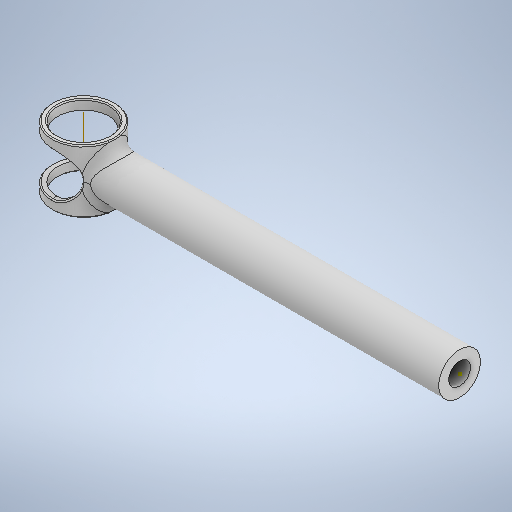
# Autodesk Inventor part: female_leg
Saved by Autodesk Inventor 2025.1 (Build 291241000, 241)
## iProperties
Created: 2024-10-31
Part Number: female_leg
Material: Generisch
Document SubType Name: Modeling
Designer: ZOMBULLI
Density: 1 g/cm^3
Appearance: Vorgabe
Author: ZOMBULLI
Autodesk Inventor part; units mm, degrees
ref_plane "YZ Plane" through (0, 0, 0) normal (1, 0, 0) x (0, 1, 0)
ref_plane "XZ Plane" through (0, 0, 0) normal (0, 1, 0) x (-1, 0, 0)
ref_plane "XY Plane" through (0, 0, 0) normal (0, 0, 1) x (1, 0, 0)
sketch "Skizze1" plane through (0, 0, 0) normal (0, 0, 1) x (1, 0, 0)
  line L0 (-34.5, 4) -> (37.5, 4)
  line L1 (37.5, 4) -> (37.5, 0)
  line L2 (37.5, 0) -> (-34.5, 0)
  line L3 (-34.5, 0) -> (-34.5, 4)
  line L4 (-48.9, 0) -> (51.9, 0) projected
  line L5 (0, 4.8) -> (0, -0.8) projected
  point P0 (0, 0)
  dimension "d0" = 72
  dimension "d1" = 4
  dimension "d2" = 0
  dimension "d3" = 37.5
  constraints: 8 end point, 2 parallel, 1 horizontal, 1 perpendicular
  measures "d0" distance of L0.start L0.end
  measures "d1" distance of L0.end L1.end
  measures "d2" distance between parallel lines of L4 L2
  measures "d3" distance between parallel lines of L1 L5
revolve "Umdrehung1" add sketch "Skizze1" angle 360 about axis through (37.5, 0, 0) along (-1, 0, 0)
sketch "Skizze2" plane through (0, 0, 0) normal (0, 0, 1) x (1, 0, 0)
  line L0 (-34.5, 4) -> (-34.5, -4) projected
  circle A0 centre (-34.5, 0) radius 6
  point P0 (0, 0)
  dimension "d5" = 12
  constraints: 1 centre point, 1 midpoint
  measures "d5" diameter of A0
extrude "Extrusion1" add sketch "Skizze2" along normal mid plane 12
fillet "Rundung1" radius 2 4 edges at (-29.3185, 3.0252, -2.6169) (-29.3186, -3.0255, -2.6166) (-29.3185, -3.0252, 2.6169) (-29.3185, 3.0252, 2.6169)
sketch "Skizze3" plane through (-34.5, 0, 6) normal (0, 0, 1) x (1, 0, 0)
  circle A0 centre (0, 0) radius 5
  point P0 (34.5, 0)
  dimension "d9" = 10
  constraints: 1 centre point
  measures "d9" diameter of A0
extrude "Extrusion2" cut sketch "Skizze3" against normal blind 15
sketch "Skizze4" plane through (0, 0, 0) normal (0, 1, 0) x (-1, 0, 0)
  line L0 (44.65, -4.15) -> (34.65, -4.15)
  line L1 (34.65, 4.15) -> (44.65, 4.15)
  line L2 (44.65, 4.15) -> (44.65, -4.15)
  arc A0 (30.5, 0) -> (34.65, -4.15) centre (34.65, 0) ccw
  arc A1 (34.65, 4.15) -> (30.5, 0) centre (34.65, 0) ccw
  line L3 (-53.715, 0) -> (59.79, 0) projected
  line L4 (30.5, 0) -> (30.5, -4.9478) construction
  line L5 (59.79, 0) -> (-53.715, 0) projected
  line L6 (29.5, 6) -> (39.5, 6) projected
  line L7 (29.5, 6) -> (29.5, -6.3947) construction
  point P0 (0, 0)
  point P1 (30.5, -2.4739)
  point P2 (30.5, 0)
  dimension "d12" = 4.15
  dimension "d13" = 8.3
  dimension "d14" = 4.15
  dimension "d15" = 1
  dimension "d16" = 10
  constraints: 10 end point, 4 point on circle, 3 vertical, 2 centre point, 2 horizontal, 2 parallel, 2 tangent, 1 coincident, 1 concentric, 1 midpoint, 1 perpendicular, 4 other
  measures "d12" radius of A0
  measures "d13" distance between parallel lines of L1 L0
  measures "d14" distance between parallel lines of L3 L0
  measures "d15" distance from line of L7 point (30.5, -2.474)
  measures "d16" distance from line of A0.centre L2
extrude "Extrusion3" cut sketch "Skizze4" along normal mid plane 15
fillet "Rundung2" radius 0.2 10 edges at (-31.6491, 5.2794, -2.8665) (-31.6485, 5.2791, 2.866) (-40.5, 0, 4.15) (-31.6491, -5.2794, -2.8665) (-31.6485, -5.2791, 2.866) (-40.5, 0, -4.15) (-40.5, 0, -6) (-39.5, 0, -6) (-39.5, 0, 6) (-40.5, 0, 6)
sketch "Skizze5" plane through (37.5, 0, 0) normal (1, 0, 0) x (0, 0, -1)
  point P0 (0, 0)
sketch "Skizze6" plane through (37.5, 0, 0) normal (1, 0, 0) x (0, 0, -1)
  circle A0 centre (0, 0) radius 2.1
  point P0 (0, 0)
  dimension "d20" = 4.2
  constraints: 1 centre point, 1 coincident
  measures "d20" diameter of A0
extrude "Extrusion4" cut sketch "Skizze6" against normal blind 4.1
